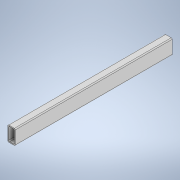
# Autodesk Inventor part: O channel 21 inch
Saved by Autodesk Inventor 2020 (Build 240168000, 168)
## iProperties
Created: 2020-02-24
Part Number: O channel 21 inch
Material: Generic
Document SubType Name: Modeling
Designer: 329817
Density: 1 g/cm^3
Appearance: Default
Author: 329817
Autodesk Inventor part; units mm, degrees
ref_plane "YZ Plane" through (0, 0, 0) normal (1, 0, 0) x (0, 1, 0)
ref_plane "XZ Plane" through (0, 0, 0) normal (0, 1, 0) x (-1, 0, 0)
ref_plane "XY Plane" through (0, 0, 0) normal (0, 0, 1) x (1, 0, 0)
sketch "Sketch1" plane through (0, 0, 0) normal (0, 0, 1) x (1, 0, 0)
  line L0 (3.175, 0) -> (22.225, 0)
  line L1 (25.4, 3.175) -> (25.4, 47.625)
  line L2 (22.225, 50.8) -> (3.175, 50.8)
  line L3 (0, 47.625) -> (0, 3.175)
  arc A0 (3.175, 50.8) -> (0, 47.625) centre (3.175, 47.625) ccw
  arc A1 (25.4, 47.625) -> (22.225, 50.8) centre (22.225, 47.625) ccw
  arc A2 (22.225, 0) -> (25.4, 3.175) centre (22.225, 3.175) ccw
  arc A3 (0, 3.175) -> (3.175, 0) centre (3.175, 3.175) ccw
  line L4 (6.35, 47.625) -> (19.05, 47.625)
  line L5 (22.225, 44.45) -> (22.225, 6.35)
  line L6 (19.05, 3.175) -> (6.35, 3.175)
  line L7 (3.175, 6.35) -> (3.175, 44.45)
  arc A4 (6.35, 47.625) -> (3.175, 44.45) centre (6.35, 44.45) ccw
  arc A5 (22.225, 44.45) -> (19.05, 47.625) centre (19.05, 44.45) ccw
  arc A6 (3.175, 6.35) -> (6.35, 3.175) centre (6.35, 6.35) ccw
  arc A7 (19.05, 3.175) -> (22.225, 6.35) centre (19.05, 6.35) ccw
  point P0 (0, 0)
  point P1 (25.4, 0)
  point P2 (0, 50.8)
  dimension "d0" = 50.8
  dimension "d1" = 25.4
  dimension "d2" = 3.175
  dimension "d3" = 3.175
  dimension "d4" = 3.175
  dimension "d5" = 3.175
  dimension "d6" = 3.175
  dimension "d7" = 3.175
  dimension "d8" = 3.175
  dimension "d9" = 3.175
  dimension "d10" = 3.175
  constraints: 16 end point, 16 point on circle, 16 tangent, 8 centre point, 6 point on line, 4 parallel, 2 perpendicular, 1 equal radius, 1 horizontal, 3 other
  measures "d0" distance of point (0, 50.8) point (0, 0)
  measures "d1" distance of point (0, 0) point (25.4, 0)
  measures "d2" radius of A0
  measures "d3" radius of A1
  measures "d4" radius of A3
  measures "d5" distance between parallel lines of L2 L4
  measures "d6" radius of A4
  measures "d7" radius of A5
  measures "d8" distance between parallel lines of L1 L5
  measures "d9" radius of A6
  measures "d10" radius of A7
extrude "Extrusion1" add sketch "Sketch1" along normal blind 533.4
body "Solid1"
